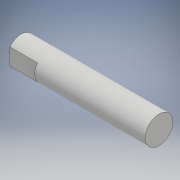
# Autodesk Inventor part: BarLimitSwitch
Saved by Autodesk Inventor 2018 (Build 220112000, 112)
## iProperties
Created: 2019-06-07
Part Number: BarLimitSwitch
Material: Generic
Document SubType Name: Modeling
Designer: aal_9
Density: 1 g/cm^3
Appearance: Default
Author: aal_9
Autodesk Inventor part; units mm, degrees
ref_plane "YZ Plane" through (0, 0, 0) normal (1, 0, 0) x (0, 1, 0)
ref_plane "XZ Plane" through (0, 0, 0) normal (0, 1, 0) x (-1, 0, 0)
ref_plane "XY Plane" through (0, 0, 0) normal (0, 0, 1) x (1, 0, 0)
sketch "Sketch1" plane through (0, 0, 0) normal (1, 0, 0) x (0, 1, 0)
  circle A0 centre (0, 0) radius 2.5
  dimension "d0" = 5
  constraints: 1 centre point, 1 coincident
  measures "d0" diameter of A0
extrude "Extrusion1" add sketch "Sketch1" along normal blind 25
sketch "Sketch2" plane through (0, 0, 0) normal (-1, 0, 0) x (0, 0, 1)
  circle A0 centre (0, 0) radius 2.5 projected
  line L0 (-1.5, -2) -> (1.9115, -2)
  line L1 (1.9115, -2) -> (1.9115, -2.5)
  line L2 (1.9115, -2.5) -> (-1.5, -2.5)
  line L3 (-1.5, -2.5) -> (-1.5, -2)
  dimension "d3" = 0.5
  constraints: 8 end point, 2 parallel, 1 horizontal, 1 perpendicular, 2 other
  measures "d3" distance of L0.end L1.end
extrude "Extrusion2" cut sketch "Sketch2" against normal blind 5 contours L0 A0 | A0 L2 L3 | L0 L1 L2 A0 picked at (0.3466, -2.0912)
body "Solid1"
